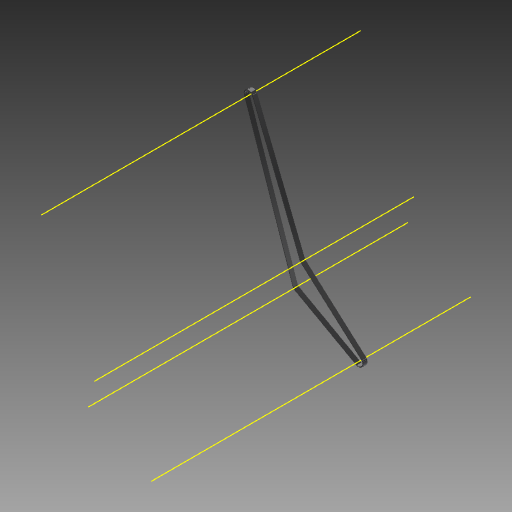
# Autodesk Inventor part: Zahnriemen
Saved by Autodesk Inventor 2019.1 (Build 231200000, 200)
## iProperties
Created: 2018-11-28
Part Number: Zahnriemen
Material: Rubber
Document SubType Name: Modeling
Designer: JochenAlt
Density: 1 g/cm^3
Appearance: Rubber - Black - Version 1.1
CustomPartVersion: 1
Author: JochenAlt
Autodesk Inventor part; units mm, degrees
ref_plane "YZ Plane" through (0, 0, 0) normal (1, 0, 0) x (0, 1, 0)
ref_plane "XZ Plane" through (0, 0, 0) normal (0, 1, 0) x (-1, 0, 0)
ref_plane "XY Plane" through (0, 0, 0) normal (0, 0, 1) x (1, 0, 0)
sketch "Skizzenpfad" plane through (0, 0, 0) normal (0, 0, 1) x (1, 0, 0)
  arc A0 (-121.993606, 18.184785) -> (-120.891175, 16.869895) centre (-119.7352, 18.958683) ccw
  arc A1 (-159.021735, 150.773441) -> (-166.47971, 148.005077) centre (-162.7157, 149.294908) ccw
  arc A2 (-115.355556, 41.677972) -> (-115.012288, 41.189389) centre (-114.148643, 42.161047) ccw
  arc A3 (-64.162842, -14.524652) -> (-59.592883, -8.069413) centre (-62.236216, -11.043338) ccw
  line L0 (-64.162842, -14.524652) -> (-120.891175, 16.869895)
  line L1 (-121.993606, 18.184785) -> (-166.47971, 148.005077)
  line L2 (-159.021735, 150.773441) -> (-115.355556, 41.677972)
  line L3 (-115.012288, 41.189389) -> (-59.592883, -8.069413)
  constraints: 8 end point, 8 point on circle, 4 centre point
ref_plane "Querschnittsebene" through (-120.891175, 16.869895, 0) normal (0.8749497, -0.4842139, 0) x (0, 0, 1)
ref_plane "Arbeitsebene2" through (-119.7352, 18.958683, 0) normal (-1, 0, 0) x (0, 0, 1)
ref_plane "Arbeitsebene3" through (-162.7157, 149.294908, 0) normal (-0.2471484, -0.9689776, 0) x (0, 0, 1)
ref_plane "Arbeitsebene4" through (-62.236216, -11.043338, 0) normal (-0.3155965, 0.9488935, 0) x (0, 0, 1)
sketch "Querschnitt" plane through (-120.891175, 16.869895, 0) normal (0.8749497, -0.4842139, 0) x (0, 0, 1)
  line L0 (-2, 0.3) -> (2, 0.3)
  line L1 (2, 0.3) -> (2, -0.3)
  line L2 (2, -0.3) -> (-2, -0.3)
  line L3 (-2, -0.3) -> (-2, 0.3)
  line L4 (-2, 0) -> (2, 0) construction
  point P0 (0, 0)
  point P1 (0, 0)
  dimension "d0" = 4
  dimension "d4" = 0.3
  dimension "d5" = 0.3
  constraints: 10 end point, 3 midpoint, 2 parallel, 1 coincident, 1 horizontal, 1 perpendicular, 1 other
  measures "d0" distance between parallel lines of L1 L3
  measures "d4" distance between parallel lines of L2 L4
  measures "d5" distance between parallel lines of L4 L0
sweep "Riemen" add profiles "Querschnitt" path "Skizzenpfad" path curves L3 A3 L0 A0 L1 A1 L2 A2
equation "\"d0\" = da_B"
equation "\"d4\" = da_a"
equation "\"d5\" = da_a2"
equation "\"da_B\" = 4"
equation "\"da_pb\" = 2.5"
equation "\"da_a\" = 0.3"
equation "\"da_S\" = 1.5"
equation "\"da_Beta\" = 20deg"
equation "\"da_Ht\" = 0.7"
equation "\"da_H\" = 1.3"
equation "\"da_a2\" = 0.3"
body "Solid1"
